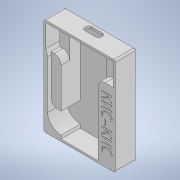
# Autodesk Inventor part: Корпус
Saved by Autodesk Inventor 2021.2 (Build 252289000, 289)
## iProperties
Created: 2023-10-18
Part Number: Корпус
Material: Типовые
Document SubType Name: Modeling
Designer: DELL
Density: 1 g/cm^3
Appearance: По умолчанию
Author: DELL
Autodesk Inventor part; units mm, degrees
ref_plane "YZ Plane" through (0, 0, 0) normal (1, 0, 0) x (0, 1, 0)
ref_plane "XZ Plane" through (0, 0, 0) normal (0, 1, 0) x (-1, 0, 0)
ref_plane "XY Plane" through (0, 0, 0) normal (0, 0, 1) x (1, 0, 0)
sketch "Эскиз1" plane through (0, 0, 0) normal (0, 0, 1) x (1, 0, 0)
  line L0 (10.25, -26.5) -> (-10.25, -26.5) construction
  line L1 (-10.25, -26.5) -> (-10.25, 26.5) construction
  line L2 (-10.25, 26.5) -> (10.25, 26.5) construction
  line L3 (10.25, 26.5) -> (10.25, -26.5) construction
  line L4 (10.25, -26.5) -> (-10.25, 26.5) construction
  line L5 (-10.25, -26.5) -> (10.25, 26.5) construction
  line L6 (19, 14.5) -> (-19, 14.5) construction
  line L7 (-19, 14.5) -> (-19, 26.5) construction
  line L8 (-19, 26.5) -> (19, 26.5) construction
  line L9 (19, 26.5) -> (19, 14.5) construction
  line L10 (19, 14.5) -> (-19, 26.5) construction
  line L11 (-19, 14.5) -> (19, 26.5) construction
  line L12 (-19.5, 14) -> (-14.75, 14)
  arc A0 (-10.75, 10) -> (-14.75, 14) centre (-14.75, 10) ccw
  line L13 (-10.75, 10) -> (-10.75, -27)
  line L14 (-10.75, -27) -> (10.75, -27)
  line L15 (10.75, -27) -> (10.75, 10)
  arc A1 (14.75, 14) -> (10.75, 10) centre (14.75, 10) ccw
  line L16 (14.75, 14) -> (19.5, 14)
  line L17 (19.5, 14) -> (19.5, 27)
  line L18 (19.5, 27) -> (-19.5, 27)
  line L19 (-19.5, 27) -> (-19.5, 14)
  line L20 (0, 26.5) -> (0, -26.5) construction
  line L21 (20.7, -28.2) -> (-20.7, -28.2)
  line L22 (-20.7, -28.2) -> (-20.7, 28.2)
  line L23 (-20.7, 28.2) -> (20.7, 28.2)
  line L24 (20.7, 28.2) -> (20.7, -28.2)
  line L25 (20.7, -28.2) -> (-20.7, 28.2) construction
  line L26 (-20.7, -28.2) -> (20.7, 28.2) construction
  line L27 (-10.75, 10) -> (-10.75, 27)
  line L28 (10.75, 10) -> (10.75, 27)
  point P0 (0, 0)
  point P1 (0, 20.5)
  point P2 (0, 20.5)
  point P3 (0, 0)
  point P4 (0, 0)
  dimension "d0" = 20.5
  dimension "d1" = 53
  dimension "d2" = 38
  dimension "d3" = 12
  dimension "d4" = 0
  dimension "d5" = 0.5
  dimension "d8" = 0.5
  dimension "d9" = 0.5
  dimension "d10" = 0.5
  dimension "d11" = 0.5
  dimension "d12" = 4
  dimension "d13" = 1.2
  dimension "d14" = 1.2
  dimension "d15" = 1.2
  constraints: 58 end point, 11 midpoint, 10 perpendicular, 7 parallel, 5 horizontal, 4 point on circle, 4 tangent, 3 point on line, 2 centre point, 1 vertical alignment, 3 other
  measures "d0" distance of L1.end L2.end
  measures "d1" distance of L0.end L1.end
  measures "d2" distance of L7.end L8.end
  measures "d3" distance of L6.end L7.end
  measures "d4" distance between parallel lines of L2 L8
  measures "d5" distance between parallel lines of L19 L7
  measures "d8" distance between parallel lines of L18 L8
  measures "d9" distance between parallel lines of L6 L12
  measures "d10" distance between parallel lines of L1 L13
  measures "d11" distance between parallel lines of L0 L14
  measures "d12" radius of A0
  measures "d13" distance between parallel lines of L23 L18
  measures "d14" distance between parallel lines of L22 L19
  measures "d15" distance between parallel lines of L14 L21
extrude "Выдавливание1" add sketch "Эскиз1" along normal blind 6 contours L19 L18 L27 A0 L12 | L18 L17 L16 A1 L28 | L21 L22 L23 L24
extrude "Выдавливание2" add sketch "Эскиз1" along normal blind 5 from surface at 6
extrude "Выдавливание3" add sketch "Эскиз1" against normal blind 1 contours L19 L18 L27 A0 L12 | L27 L18 L28 L15 L14 L13 | L18 L17 L16 A1 L28 | L21 L22 L23 L24
fillet "Сопряжение1" radius 1 4 edges at (-20.7, 28.2, 5) (20.7, 28.2, 5) (-20.7, -28.2, 5) (20.7, -28.2, 5)
chamfer "Фаска1" distance 0.5 angle 45 8 edges at (20.7, 0, -1) (20.4071, -27.9071, -1) (0, -28.2, -1) (-20.4071, -27.9071, -1) (-20.7, 0, -1) (-20.4071, 27.9071, -1) (0, 28.2, -1) (20.4071, 27.9071, -1)
sketch "Эскиз2" plane through (-19.7, 28.2, 11) normal (0, 1, 0) x (1, 0, 0)
  line L0 (8.95, 11) -> (30.45, 11) construction
  line L1 (8.95, 11) -> (8.95, 5) construction
  line L2 (30.45, 11) -> (30.45, 5) construction
  line L3 (22.7, 8) -> (16.7, 8) construction
  line L4 (22.7, 10) -> (16.7, 10)
  line L5 (16.7, 6) -> (22.7, 6)
  arc A0 (22.7, 6) -> (22.7, 10) centre (22.7, 8) ccw
  arc A1 (16.7, 10) -> (16.7, 6) centre (16.7, 8) ccw
  point P0 (19.7, 11)
  point P1 (19.7, 8)
  point P2 (19.7, 11)
  dimension "d26" = 10
  dimension "d27" = 4
  dimension "d28" = 1
  constraints: 8 end point, 4 point on circle, 4 tangent, 2 centre point, 2 midpoint, 2 parallel, 1 vertical alignment
  measures "d27" distance between parallel lines of L5 L4
  measures "d28" distance between parallel lines of L4 L0
extrude "Выдавливание4" cut sketch "Эскиз2" against normal up to next
sketch "Эскиз3" plane through (-19.7, 28.2, 11) normal (0, 0, 1) x (1, 0, 0)
  line L0 (38.4355, -18.4335) -> (38.4355, -51.3182) construction
  line L1 (38.4355, -51.3182) -> (33.2904, -51.3182) construction
  line L2 (33.2904, -51.3182) -> (33.2904, -18.4335) construction
  line L3 (33.2904, -18.4335) -> (38.4355, -18.4335) construction
  line L4 (39.4, -56.4) -> (0, -56.4) construction
  line L5 (19.7, -56.4) -> (19.7, 0) construction
  line L6 (16.7, 0) -> (22.7, 0) construction
  line L7 (35.4384, -20.4584) -> (34.6425, -19.7935)
  line L8 (34.6425, -19.7935) -> (32.7183, -19.7935)
  spline S0 degree 2 poles (32.7183, -19.7935) (32.3355, -19.7935) (32.3355, -19.4107) knots 0 0 0 1 1 1
  spline S1 degree 2 poles (32.3355, -19.4107) (32.3355, -19.0279) (32.7183, -19.0279) knots 0 0 0 1 1 1
  line L9 (32.7183, -19.0279) -> (38.0577, -19.0279)
  spline S2 degree 2 poles (38.0577, -19.0279) (38.4355, -19.0279) (38.4355, -19.4107) knots 0 0 0 1 1 1
  spline S3 degree 2 poles (38.4355, -19.4107) (38.4355, -19.7935) (38.0577, -19.7935) knots 0 0 0 1 1 1
  line L10 (38.0577, -19.7935) -> (35.65, -19.7935)
  line L11 (35.65, -19.7935) -> (38.3096, -22.0905)
  spline S4 degree 2 poles (38.3096, -22.0905) (38.4355, -22.2013) (38.4355, -22.3776) knots 0 0 0 1 1 1
  spline S5 degree 2 poles (38.4355, -22.3776) (38.4355, -22.7604) (38.0577, -22.7604) knots 0 0 0 1 1 1
  spline S6 degree 2 poles (38.0577, -22.7604) (37.9116, -22.7604) (37.7706, -22.5338) knots 0 0 0 1 1 1
  line L12 (37.7706, -22.5338) -> (35.9774, -20.9823)
  line L13 (35.9774, -20.9823) -> (32.9047, -22.705)
  spline S7 degree 2 poles (32.9047, -22.705) (32.814, -22.7604) (32.7183, -22.7604) knots 0 0 0 1 1 1
  spline S8 degree 2 poles (32.7183, -22.7604) (32.5672, -22.7604) (32.3355, -22.5237) (32.3355, -22.3776) knots 0 0 0 1 2 2 2
  spline S9 degree 2 poles (32.3355, -22.3776) (32.3355, -22.1459) (32.5823, -22.025) knots 0 0 0 1 1 1
  line L14 (32.5823, -22.025) -> (35.4384, -20.4584)
  spline S10 degree 2 poles (38.4355, -27.1226) (38.4355, -27.5054) (38.0577, -27.5054) knots 0 0 0 1 1 1
  line L15 (38.0577, -27.5054) -> (32.7183, -27.5054)
  spline S11 degree 2 poles (32.7183, -27.5054) (32.3355, -27.5054) (32.3355, -27.1226) knots 0 0 0 1 1 1
  spline S12 degree 2 poles (32.3355, -27.1226) (32.3355, -26.7398) (32.7183, -26.7398) knots 0 0 0 1 1 1
  line L16 (32.7183, -26.7398) -> (36.5869, -26.7398)
  line L17 (36.5869, -26.7398) -> (32.9903, -24.5436)
  spline S13 degree 2 poles (32.9903, -24.5436) (32.6881, -24.5436) (32.5874, -24.5134) knots 0 0 0 1 1 1
  spline S14 degree 2 poles (32.5874, -24.5134) (32.3355, -24.4479) (32.3355, -24.1608) knots 0 0 0 1 1 1
  spline S15 degree 2 poles (32.3355, -24.1608) (32.3355, -23.7779) (32.7183, -23.7779) knots 0 0 0 1 1 1
  line L18 (32.7183, -23.7779) -> (38.0577, -23.7779)
  spline S16 degree 2 poles (38.0577, -23.7779) (38.4355, -23.7779) (38.4355, -24.1608) knots 0 0 0 1 1 1
  spline S17 degree 2 poles (38.4355, -24.1608) (38.4355, -24.5436) (38.0577, -24.5436) knots 0 0 0 1 1 1
  line L19 (38.0577, -24.5436) -> (34.1892, -24.5436)
  line L20 (34.1892, -24.5436) -> (37.7857, -26.7398)
  spline S18 degree 2 poles (37.7857, -26.7398) (38.0879, -26.7398) (38.1836, -26.765) knots 0 0 0 1 1 1
  spline S19 degree 2 poles (38.1836, -26.765) (38.4355, -26.8305) (38.4355, -27.1226) knots 0 0 0 1 1 1
  spline S20 degree 2 poles (38.4355, -31.2833) (38.4355, -31.6661) (38.0577, -31.6661) knots 0 0 0 1 1 1
  spline S21 degree 2 poles (38.0577, -31.6661) (37.6749, -31.6661) (37.6749, -31.2833) knots 0 0 0 1 1 1
  line L21 (37.6749, -31.2833) -> (37.6749, -30.0996)
  spline S22 degree 2 poles (37.6749, -30.0996) (37.6749, -29.6362) (37.277, -29.4044) knots 0 0 0 1 1 1
  spline S23 degree 2 poles (37.277, -29.4044) (37.0906, -29.2936) (36.8689, -29.2936) knots 0 0 0 1 1 1
  line L22 (36.8689, -29.2936) -> (33.9071, -29.2936)
  spline S24 degree 2 poles (33.9071, -29.2936) (33.5696, -29.2936) (33.0961, -29.7671) (33.0961, -30.0996) knots 0 0 0 1 2 2 2
  line L23 (33.0961, -30.0996) -> (33.0961, -31.2833)
  spline S25 degree 2 poles (33.0961, -31.2833) (33.0961, -31.6661) (32.7183, -31.6661) knots 0 0 0 1 1 1
  spline S26 degree 2 poles (32.7183, -31.6661) (32.3355, -31.6661) (32.3355, -31.2833) knots 0 0 0 1 1 1
  line L24 (32.3355, -31.2833) -> (32.3355, -30.0996)
  spline S27 degree 2 poles (32.3355, -30.0996) (32.3355, -29.4447) (33.2523, -28.528) (33.9071, -28.528) knots 0 0 0 1 2 2 2
  line L25 (33.9071, -28.528) -> (36.874, -28.528)
  spline S28 degree 2 poles (36.874, -28.528) (37.5187, -28.528) (38.4355, -29.4447) (38.4355, -30.0996) knots 0 0 0 1 2 2 2
  line L26 (38.4355, -30.0996) -> (38.4355, -31.2833)
  line L27 (33.8164, -35.439) -> (33.8164, -33.0665)
  spline S29 degree 2 poles (33.8164, -33.0665) (33.8164, -32.6836) (34.1993, -32.6836) knots 0 0 0 1 1 1
  spline S30 degree 2 poles (34.1993, -32.6836) (34.577, -32.6836) (34.577, -33.0665) knots 0 0 0 1 1 1
  line L28 (34.577, -33.0665) -> (34.577, -35.439)
  spline S31 degree 2 poles (34.577, -35.439) (34.577, -35.8218) (34.1993, -35.8218) knots 0 0 0 1 1 1
  spline S32 degree 2 poles (34.1993, -35.8218) (33.8164, -35.8218) (33.8164, -35.439) knots 0 0 0 1 1 1
  line L29 (35.4384, -38.2698) -> (34.6425, -37.6049)
  line L30 (34.6425, -37.6049) -> (32.7183, -37.6049)
  spline S33 degree 2 poles (32.7183, -37.6049) (32.3355, -37.6049) (32.3355, -37.2221) knots 0 0 0 1 1 1
  spline S34 degree 2 poles (32.3355, -37.2221) (32.3355, -36.8393) (32.7183, -36.8393) knots 0 0 0 1 1 1
  line L31 (32.7183, -36.8393) -> (38.0577, -36.8393)
  spline S35 degree 2 poles (38.0577, -36.8393) (38.4355, -36.8393) (38.4355, -37.2221) knots 0 0 0 1 1 1
  spline S36 degree 2 poles (38.4355, -37.2221) (38.4355, -37.6049) (38.0577, -37.6049) knots 0 0 0 1 1 1
  line L32 (38.0577, -37.6049) -> (35.65, -37.6049)
  line L33 (35.65, -37.6049) -> (38.3096, -39.9019)
  spline S37 degree 2 poles (38.3096, -39.9019) (38.4355, -40.0127) (38.4355, -40.189) knots 0 0 0 1 1 1
  spline S38 degree 2 poles (38.4355, -40.189) (38.4355, -40.5718) (38.0577, -40.5718) knots 0 0 0 1 1 1
  spline S39 degree 2 poles (38.0577, -40.5718) (37.9116, -40.5718) (37.7706, -40.3452) knots 0 0 0 1 1 1
  line L34 (37.7706, -40.3452) -> (35.9774, -38.7937)
  line L35 (35.9774, -38.7937) -> (32.9047, -40.5164)
  spline S40 degree 2 poles (32.9047, -40.5164) (32.814, -40.5718) (32.7183, -40.5718) knots 0 0 0 1 1 1
  spline S41 degree 2 poles (32.7183, -40.5718) (32.5672, -40.5718) (32.3355, -40.3351) (32.3355, -40.189) knots 0 0 0 1 2 2 2
  spline S42 degree 2 poles (32.3355, -40.189) (32.3355, -39.9573) (32.5823, -39.8364) knots 0 0 0 1 1 1
  line L36 (32.5823, -39.8364) -> (35.4384, -38.2698)
  spline S43 degree 2 poles (38.4355, -44.934) (38.4355, -45.3168) (38.0577, -45.3168) knots 0 0 0 1 1 1
  line L37 (38.0577, -45.3168) -> (32.7183, -45.3168)
  spline S44 degree 2 poles (32.7183, -45.3168) (32.3355, -45.3168) (32.3355, -44.934) knots 0 0 0 1 1 1
  spline S45 degree 2 poles (32.3355, -44.934) (32.3355, -44.5512) (32.7183, -44.5512) knots 0 0 0 1 1 1
  line L38 (32.7183, -44.5512) -> (36.5869, -44.5512)
  line L39 (36.5869, -44.5512) -> (32.9903, -42.355)
  spline S46 degree 2 poles (32.9903, -42.355) (32.6881, -42.355) (32.5874, -42.3248) knots 0 0 0 1 1 1
  spline S47 degree 2 poles (32.5874, -42.3248) (32.3355, -42.2593) (32.3355, -41.9722) knots 0 0 0 1 1 1
  spline S48 degree 2 poles (32.3355, -41.9722) (32.3355, -41.5893) (32.7183, -41.5893) knots 0 0 0 1 1 1
  line L40 (32.7183, -41.5893) -> (38.0577, -41.5893)
  spline S49 degree 2 poles (38.0577, -41.5893) (38.4355, -41.5893) (38.4355, -41.9722) knots 0 0 0 1 1 1
  spline S50 degree 2 poles (38.4355, -41.9722) (38.4355, -42.355) (38.0577, -42.355) knots 0 0 0 1 1 1
  line L41 (38.0577, -42.355) -> (34.1892, -42.355)
  line L42 (34.1892, -42.355) -> (37.7857, -44.5512)
  spline S51 degree 2 poles (37.7857, -44.5512) (38.0879, -44.5512) (38.1836, -44.5764) knots 0 0 0 1 1 1
  spline S52 degree 2 poles (38.1836, -44.5764) (38.4355, -44.6419) (38.4355, -44.934) knots 0 0 0 1 1 1
  spline S53 degree 2 poles (38.4355, -49.0947) (38.4355, -49.4775) (38.0577, -49.4775) knots 0 0 0 1 1 1
  spline S54 degree 2 poles (38.0577, -49.4775) (37.6749, -49.4775) (37.6749, -49.0947) knots 0 0 0 1 1 1
  line L43 (37.6749, -49.0947) -> (37.6749, -47.911)
  spline S55 degree 2 poles (37.6749, -47.911) (37.6749, -47.4475) (37.277, -47.2158) knots 0 0 0 1 1 1
  spline S56 degree 2 poles (37.277, -47.2158) (37.0906, -47.105) (36.8689, -47.105) knots 0 0 0 1 1 1
  line L44 (36.8689, -47.105) -> (33.9071, -47.105)
  spline S57 degree 2 poles (33.9071, -47.105) (33.5696, -47.105) (33.0961, -47.5785) (33.0961, -47.911) knots 0 0 0 1 2 2 2
  line L45 (33.0961, -47.911) -> (33.0961, -49.0947)
  spline S58 degree 2 poles (33.0961, -49.0947) (33.0961, -49.4775) (32.7183, -49.4775) knots 0 0 0 1 1 1
  spline S59 degree 2 poles (32.7183, -49.4775) (32.3355, -49.4775) (32.3355, -49.0947) knots 0 0 0 1 1 1
  line L46 (32.3355, -49.0947) -> (32.3355, -47.911)
  spline S60 degree 2 poles (32.3355, -47.911) (32.3355, -47.2561) (33.2523, -46.3394) (33.9071, -46.3394) knots 0 0 0 1 2 2 2
  line L47 (33.9071, -46.3394) -> (36.874, -46.3394)
  spline S61 degree 2 poles (36.874, -46.3394) (37.5187, -46.3394) (38.4355, -47.2561) (38.4355, -47.911) knots 0 0 0 1 2 2 2
  line L48 (38.4355, -47.911) -> (38.4355, -49.0947)
  point P0 (19.7, -28.2)
  constraints: 2 end point, 2 midpoint, 2 other
emboss "Рельеф1" sketch "Эскиз3" operation cut depth 0.6 direction (0, 0, -1)
sketch "Эскиз4" plane through (-19.7, 28.2, 11) normal (0, 0, 1) x (1, 0, 0)
  line L0 (8.95, -18.2) -> (8.95, -55.2) construction
  line L1 (0.2, -1.2) -> (0.2, -14.2) construction
  line L2 (0.2, -1.2) -> (3.2, -1.2)
  line L3 (8.95, -1.2) -> (0.2, -1.2) construction
  line L4 (3.2, -1.2) -> (3.2, -14.2)
  line L5 (0.2, -14.2) -> (4.95, -14.2) construction
  line L6 (0.2, -14.2) -> (3.2, -14.2) construction
  line L7 (0.2, -14.2) -> (0.2, -1.2)
  line L8 (8.95, -55.2) -> (30.45, -55.2) construction
  line L9 (1.2, -17.8192) -> (1.2, -45.7113)
  line L10 (3.2, -37.8219) -> (3.2, -14.2)
  line L11 (1.2, -17.8192) -> (1.2, -16.0429) construction
  line L12 (1.2, -16.0429) -> (0.2, -15.3575) construction
  line L13 (0.2, -15.3575) -> (0.2, -14.2) construction
  spline S0 degree 3 poles (1.2, -17.8192) (1.2, -16.0429) (0.2, -15.3575) (0.2, -14.2) knots 1 1 1 1 2 2 2 2
  line L14 (8.95, -53.2) -> (3.0919, -52.2989) construction
  line L15 (3.0919, -52.2989) -> (1.2, -48.7736) construction
  line L16 (1.2, -48.7736) -> (1.2, -45.7113) construction
  spline S1 degree 3 poles (8.95, -53.2) (3.0919, -52.2989) (1.2, -48.7736) (1.2, -45.7113) knots 1 1 1 1 2 2 2 2
  line L17 (8.95, -41.2) -> (4.9393, -41.2) construction
  line L18 (4.9393, -41.2) -> (3.2, -39.7886) construction
  line L19 (3.2, -39.7886) -> (3.2, -37.8219) construction
  spline S2 degree 3 poles (8.95, -41.2) (4.9393, -41.2) (3.2, -39.7886) (3.2, -37.8219) knots 1 1 1 1 2 2 2 2
  line L20 (8.95, -53.2) -> (8.95, -41.2)
  point P0 (19.7, -28.2)
  dimension "d34" = 3
  dimension "d37" = 2
  dimension "d38" = 12
  dimension "d39" = 2
  constraints: 14 end point, 5 point on line, 5 vertical, 3 perpendicular, 1 collinear, 1 horizontal, 9 other
  measures "d34" distance of L1.start L2.end
  measures "d37" distance from line of L14.start L8
  measures "d38" distance of L17.start L14.start
  measures "d39" distance between parallel lines of L9 L10
extrude "Выдавливание5" cut sketch "Эскиз4" against normal up to surface (11 mm away)
equation "\"d8\" = d5"
equation "\"d9\" = d5"
equation "\"d10\" = d5"
equation "\"d11\" = d5"
equation "\"d14\" = d13"
equation "\"d15\" = d13"
